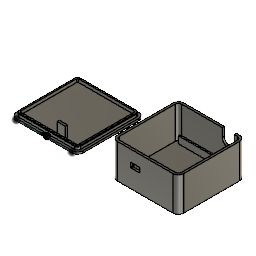
dtu-case-fusion360-archive (Autodesk Fusion 360 design; units mm, degrees)
Autodesk Fusion 360 part; units mm, degrees
sketch "Skizze1" plane through (0, 0, 0) normal (0, 0, 1) x (1, 0, 0)
  line L0 (4.346, 49.2651) -> (56.346, 49.2651)
  line L1 (61.346, 44.2651) -> (61.346, -7.7349)
  line L2 (56.346, -12.7349) -> (4.346, -12.7349)
  line L3 (-0.654, -7.7349) -> (-0.654, 44.2651)
  arc A0 (4.346, 49.2651) -> (-0.654, 44.2651) centre (4.346, 44.2651) ccw
  arc A1 (61.346, 44.2651) -> (56.346, 49.2651) centre (56.346, 44.2651) ccw
  arc A2 (56.346, -12.7349) -> (61.346, -7.7349) centre (56.346, -7.7349) ccw
  arc A3 (-0.654, -7.7349) -> (4.346, -12.7349) centre (4.346, -7.7349) ccw
  arc A4 (59.346, 44.2651) -> (56.346, 47.2651) centre (56.346, 44.2651) ccw
  line L4 (4.346, 47.2651) -> (56.346, 47.2651)
  arc A5 (4.346, 47.2651) -> (1.346, 44.2651) centre (4.346, 44.2651) ccw
  line L5 (1.346, -7.7349) -> (1.346, 44.2651)
  arc A6 (1.346, -7.7349) -> (4.346, -10.7349) centre (4.346, -7.7349) ccw
  line L6 (56.346, -10.7349) -> (4.346, -10.7349)
  arc A7 (56.346, -10.7349) -> (59.346, -7.7349) centre (56.346, -7.7349) ccw
  line L7 (59.346, 44.2651) -> (59.346, -7.7349)
  point P0 (-0.654, 49.2651)
  point P1 (61.346, 49.2651)
  point P2 (-0.654, -12.7349)
  dimension "d1" = 62
  dimension "d2" = 62
  dimension "d3" = 5
  dimension "d4" = 5
  dimension "d5" = 2
  constraint horizontal L0
  constraint vertical L1
  constraint horizontal L2
  constraint vertical L3
  constraint coincident P0 L0
  constraint coincident P0 L3
  constraint tangent L0 A0
  constraint tangent L3 A0
  constraint coincident P1 L0
  constraint coincident P1 L1
  constraint tangent L0 A1
  constraint tangent L1 A1
  constraint tangent L1 A2
  constraint tangent L2 A2
  constraint equal A1 A2
  constraint coincident P2 L2
  constraint coincident P2 L3
  constraint tangent L2 A3
  constraint tangent L3 A3
  constraint equal A1 A3
  measures "d1" distance of P0 P1
  measures "d2" distance of P0 P2
  measures "d3" radius of A0
  measures "d4" radius of A1
extrude "Extrusion1" add sketch "Skizze1" along normal blind 2 contours A4 L4 A5 L5 A6 L6 A7 L7 makes body 1
extrude "Extrusion2" add sketch "Skizze1" along normal blind 32 bodies 1
sketch "Skizze2" plane through (0, 0, 2) normal (0, 0, 1) x (-1, 0, 0)
  arc A0 (-4.346, -47.2651) -> (-1.346, -44.2651) centre (-4.346, -44.2651) ccw
  line L0 (-1.346, -44.2651) -> (-1.346, 7.7349)
  arc A1 (-1.346, 7.7349) -> (-4.346, 10.7349) centre (-4.346, 7.7349) ccw
  line L1 (-4.346, 10.7349) -> (-56.346, 10.7349)
  arc A2 (-56.346, 10.7349) -> (-59.346, 7.7349) centre (-56.346, 7.7349) ccw
  line L2 (-59.346, 7.7349) -> (-59.346, -44.2651)
  arc A3 (-59.346, -44.2651) -> (-56.346, -47.2651) centre (-56.346, -44.2651) ccw
  line L3 (-56.346, -47.2651) -> (-4.346, -47.2651)
  line L4 (-30.346, -44.2651) -> (-30.346, 7.7349) construction
  line L5 (-55.846, 7.2349) -> (-4.846, 7.2349)
  line L6 (-4.846, -43.7651) -> (-55.846, -43.7651)
  line L7 (-55.846, 7.2349) -> (-4.846, -43.7651) construction
  line L8 (-4.846, 7.2349) -> (-55.846, -43.7651) construction
  line L9 (-47.726, -43.7651) -> (-47.726, 7.2349) construction
  line L10 (-4.846, -28.7651) -> (-55.846, -28.7651) construction
  circle A4 centre (-47.726, -28.7651) radius 1.5
  line L11 (-13.846, 7.2349) -> (-13.846, -43.7651) construction
  line L12 (-22.846, 7.2349) -> (-22.846, -43.7651) construction
  line L13 (-55.846, -43.7651) -> (-55.846, -45.2651)
  line L14 (-4.846, -43.7651) -> (-4.846, -45.2651)
  line L15 (-4.846, -45.2651) -> (-55.846, -45.2651)
  line L16 (-4.846, 7.2349) -> (-4.846, 8.7349)
  line L17 (-55.846, 7.2349) -> (-55.846, 8.7349)
  line L18 (-4.846, 8.7349) -> (-55.846, 8.7349)
  point P0 (-30.346, -18.2651)
  dimension "d10" = -29
  dimension "d11" = 51
  dimension "d12" = 51
  dimension "d17" = 15
  dimension "d18" = 3
  dimension "d50" = 1.5
  dimension "d51" = 1.5
  dimension "d52" = 1.5
  dimension "d53" = 1.5
  constraint horizontal L5
  constraint parallel L5 L6
  constraint coincident L7 P0
  constraint coincident L8 P0
  constraint midpoint L4 P0
  constraint coincident L10 A4.centre
  constraint coincident L9 A4.centre
  constraint perpendicular L6 L13
  constraint perpendicular L6 L14
  constraint perpendicular L1 L16
  constraint perpendicular L5 L17
  measures "d11" distance of L6.start L6.end
  measures "d12" distance of L5.end L6.start
  measures "d18" diameter of A4
  measures "d50" distance of L6.end L13.end
  measures "d51" distance of L6.start L14.end
  measures "d52" distance of L5.end L16.end
  measures "d53" distance of L5.start L17.end
extrude "Extrusion4" add sketch "Skizze2" along normal blind 14 contours A4 bodies 1
sketch "Skizze4" plane through (0, 49.2651, 0) normal (0, 1, 0) x (-1, 0, 0)
  line L0 (-56.346, 0) -> (-4.346, 0)
  line L1 (-4.346, 0) -> (-4.346, 32)
  line L2 (-4.346, 32) -> (-56.346, 32)
  line L3 (-56.346, 32) -> (-56.346, 0)
  line L4 (-47.7215, 1.9893) -> (-47.7215, 32) construction
  line L5 (-56.346, 2) -> (-4.346, 2) construction
  line L6 (-56.346, 24) -> (-4.346, 24) construction
  circle A0 centre (-47.7215, 24) radius 5.5
  line L7 (-42.2215, 24) -> (-42.2215, 32)
  line L8 (-53.2215, 24) -> (-53.2215, 32)
  dimension "d21" = -2
  dimension "d22" = -24
  dimension "d23" = 11
  constraint coincident L2 L4.end
  constraint perpendicular L2 L4
  constraint coincident L6 A0.centre
  constraint coincident L4 A0.centre
  constraint coincident A0 L7.start
  constraint coincident L6 L7.start
  constraint coincident L2 L7.end
  constraint tangent A0 L7
  constraint coincident A0 L8.start
  constraint coincident L6 L8.start
  constraint coincident L2 L8.end
  constraint tangent A0 L8
  measures "d23" diameter of A0
extrude "Extrusion6" cut sketch "Skizze4" against normal blind 4 contours L2 A0 L7 L8 | A0 bodies 1
sketch "Skizze5" plane through (0, -12.7349, 0) normal (0, -1, 0) x (1, 0, 0)
  line L0 (4.346, 0) -> (56.346, 0)
  line L1 (56.346, 0) -> (56.346, 32)
  line L2 (56.346, 32) -> (4.346, 32)
  line L3 (4.346, 32) -> (4.346, 0)
  line L4 (56.346, 21.5) -> (4.346, 21.5) construction
  line L5 (56.346, 17) -> (4.346, 17) construction
  line L6 (16.846, 32) -> (16.846, 0) construction
  line L7 (25.346, 32) -> (25.346, 0) construction
  line L8 (17.346, 21.5) -> (24.846, 21.5)
  line L9 (25.346, 21) -> (25.346, 17.5)
  line L10 (24.846, 17) -> (17.346, 17)
  line L11 (16.846, 17.5) -> (16.846, 21)
  arc A0 (17.346, 21.5) -> (16.846, 21) centre (17.346, 21) ccw
  arc A1 (25.346, 21) -> (24.846, 21.5) centre (24.846, 21) ccw
  arc A2 (24.846, 17) -> (25.346, 17.5) centre (24.846, 17.5) ccw
  arc A3 (16.846, 17.5) -> (17.346, 17) centre (17.346, 17.5) ccw
  dimension "d58" = -10.5
  dimension "d59" = -15
  dimension "d60" = -12.5
  dimension "d61" = -21
  dimension "d62" = 0.5
  constraint horizontal L8
  constraint vertical L9
  constraint horizontal L10
  constraint vertical L11
  constraint tangent L8 A0
  constraint tangent L11 A0
  constraint tangent L8 A1
  constraint tangent L9 A1
  constraint equal A0 A1
  constraint tangent L9 A2
  constraint tangent L10 A2
  constraint equal A0 A2
  constraint tangent L10 A3
  constraint tangent L11 A3
  constraint equal A0 A3
  measures "d62" radius of A0
sketch "Skizze6" plane through (0, 0, 0) normal (0, 0, 1) x (1, 0, 0)
  line L0 (-91.052, 50.8088) -> (-39.052, 50.8088)
  line L1 (-34.052, 45.8088) -> (-34.052, -6.1912)
  line L2 (-39.052, -11.1912) -> (-91.052, -11.1912)
  line L3 (-96.052, -6.1912) -> (-96.052, 45.8088)
  arc A0 (-91.052, 50.8088) -> (-96.052, 45.8088) centre (-91.052, 45.8088) ccw
  arc A1 (-34.052, 45.8088) -> (-39.052, 50.8088) centre (-39.052, 45.8088) ccw
  arc A2 (-39.052, -11.1912) -> (-34.052, -6.1912) centre (-39.052, -6.1912) ccw
  arc A3 (-96.052, -6.1912) -> (-91.052, -11.1912) centre (-91.052, -6.1912) ccw
  arc A4 (-91.052, 48.6788) -> (-93.922, 45.8088) centre (-91.052, 45.8088) ccw
  line L4 (-93.922, -6.1912) -> (-93.922, 45.8088)
  arc A5 (-93.922, -6.1912) -> (-91.052, -9.0612) centre (-91.052, -6.1912) ccw
  line L5 (-39.052, -9.0612) -> (-91.052, -9.0612)
  arc A6 (-39.052, -9.0612) -> (-36.182, -6.1912) centre (-39.052, -6.1912) ccw
  line L6 (-36.182, 45.8088) -> (-36.182, -6.1912)
  arc A7 (-36.182, 45.8088) -> (-39.052, 48.6788) centre (-39.052, 45.8088) ccw
  line L7 (-91.052, 48.6788) -> (-39.052, 48.6788)
  arc A8 (-91.052, 46.7088) -> (-91.952, 45.8088) centre (-91.052, 45.8088) ccw
  line L8 (-91.952, -6.1912) -> (-91.952, 45.8088)
  arc A9 (-91.952, -6.1912) -> (-91.052, -7.0912) centre (-91.052, -6.1912) ccw
  line L9 (-39.052, -7.0912) -> (-91.052, -7.0912)
  arc A10 (-39.052, -7.0912) -> (-38.152, -6.1912) centre (-39.052, -6.1912) ccw
  line L10 (-38.152, 45.8088) -> (-38.152, -6.1912)
  arc A11 (-38.152, 45.8088) -> (-39.052, 46.7088) centre (-39.052, 45.8088) ccw
  line L11 (-91.052, 46.7088) -> (-39.052, 46.7088)
  line L12 (-78.952, -5.1912) -> (-71.452, -5.1912)
  line L13 (-71.452, -5.1912) -> (-71.452, -3.1912)
  line L14 (-71.452, -3.1912) -> (-78.952, -3.1912)
  line L15 (-78.952, -3.1912) -> (-78.952, -5.1912)
  point P0 (-96.052, 50.8088)
  point P1 (-34.052, 50.8088)
  point P2 (-96.052, -11.1912)
  dimension "d35" = 62
  dimension "d36" = 62
  dimension "d37" = 5
  dimension "d38" = 2.13
  dimension "d39" = 4.1
  dimension "d67" = 7.5
  dimension "d68" = 2
  constraint horizontal L0
  constraint vertical L1
  constraint horizontal L2
  constraint vertical L3
  constraint coincident P0 L0
  constraint coincident P0 L3
  constraint tangent L0 A0
  constraint tangent L3 A0
  constraint coincident P1 L0
  constraint coincident P1 L1
  constraint tangent L0 A1
  constraint tangent L1 A1
  constraint equal A0 A1
  constraint tangent L1 A2
  constraint tangent L2 A2
  constraint equal A0 A2
  constraint coincident P2 L2
  constraint coincident P2 L3
  constraint tangent L2 A3
  constraint tangent L3 A3
  constraint equal A0 A3
  constraint horizontal L12
  constraint vertical L13
  constraint horizontal L14
  constraint vertical L15
  measures "d35" distance of P0 P1
  measures "d36" distance of P0 P2
  measures "d37" radius of A0
  measures "d67" distance of L12.start L12.end
  measures "d68" distance of L12.start L14.end
extrude "Extrusion8" add sketch "Skizze6" along normal blind 5 separate body contours A4 L4 A5 L5 A6 L6 A7 L7 makes body 2
extrude "Extrusion9" add sketch "Skizze6" along normal blind 2 contours L0 L1 L2 L3 A0 A1 A2 A3 | A8 L8 A9 L9 A10 L10 A11 L11 | L12 L13 L14 L15 bodies 2
chamfer "Fase1" distance 0.5 angle 45 8 edges at (-93.922, 19.8088, 5) (-93.0814, -8.2206, 5) (-65.052, -9.0612, 5) (-37.0226, -8.2206, 5) (-36.182, 19.8088, 5) (-37.0226, 47.8382, 5) (-65.052, 48.6788, 5) (-93.0814, 47.8382, 5) on bodies 2
sketch "Skizze7" plane through (0, -11.1912, 0) normal (0, -1, 0) x (1, 0, 0)
  line L0 (-91.052, 0) -> (-39.052, 0)
  line L1 (-39.052, 0) -> (-39.052, 2)
  line L2 (-39.052, 2) -> (-91.052, 2)
  line L3 (-91.052, 2) -> (-91.052, 0)
  line L4 (-65.052, 2) -> (-65.052, 0) construction
  line L5 (-39.052, 1) -> (-91.052, 1) construction
  line L6 (-65.052, 1) -> (-62.552, 1)
  line L7 (-62.552, 1) -> (-62.552, 2)
  line L8 (-62.552, 2) -> (-67.552, 2)
  line L9 (-67.552, 2) -> (-67.552, 1)
  line L10 (-67.552, 1) -> (-65.052, 1)
  dimension "d45" = -1
  dimension "d46" = 2.5
  dimension "d47" = 5
  constraint midpoint L2 L4.start
  constraint midpoint L0 L4.end
  constraint midpoint L5 L6.start
  constraint parallel L5 L6
  constraint coincident L2 L7.end
  constraint perpendicular L2 L7
  constraint perpendicular L7 L8
  constraint coincident L5 L9.end
  constraint perpendicular L5 L9
  measures "d46" distance of L6.start L6.end
  measures "d47" distance of L7.end L8.end
extrude "Extrusion10" cut sketch "Skizze7" against normal blind 1 contours L2 L6 L7 L8 L9 L10 bodies 2
extrude "Extrusion11" add sketch "Skizze2" along normal blind 6.5 contours L6 L13 L14 L15 bodies 1
extrude "Extrusion12" add sketch "Skizze2" along normal blind 6.5 contours L5 L16 L17 L18 bodies 1
extrude "Extrusion13" cut sketch "Skizze5" against normal blind 6 contours L8 L9 L10 L11 A0 A1 A2 A3 bodies 1
sketch "Skizze8" plane through (0, 0, 2) normal (0, 0, 1) x (-1, 0, 0)
  arc A0 (91.952, 6.1912) -> (91.052, 7.0912) centre (91.052, 6.1912) ccw
  line L0 (91.052, 7.0912) -> (39.052, 7.0912)
  arc A1 (39.052, 7.0912) -> (38.152, 6.1912) centre (39.052, 6.1912) ccw
  line L1 (38.152, 6.1912) -> (38.152, -45.8088)
  arc A2 (38.152, -45.8088) -> (39.052, -46.7088) centre (39.052, -45.8088) ccw
  line L2 (39.052, -46.7088) -> (91.052, -46.7088)
  arc A3 (91.052, -46.7088) -> (91.952, -45.8088) centre (91.052, -45.8088) ccw
  line L3 (91.952, -45.8088) -> (91.952, 6.1912)
  line L4 (59.0191, 3.1992) -> (51.5191, 3.1992)
  line L5 (51.5191, 3.1992) -> (51.5191, 5.1992)
  line L6 (51.5191, 5.1992) -> (59.0191, 5.1992)
  line L7 (59.0191, 5.1992) -> (59.0191, 3.1992)
  dimension "d71" = 7.5
  dimension "d72" = 2
  constraint horizontal L4
  constraint vertical L5
  constraint horizontal L6
  constraint vertical L7
  measures "d71" distance of L4.start L4.end
  measures "d72" distance of L4.start L6.end
extrude "Extrusion15" add sketch "Skizze8" along normal blind 10.5 contours L4 L5 L6 L7 bodies 2
